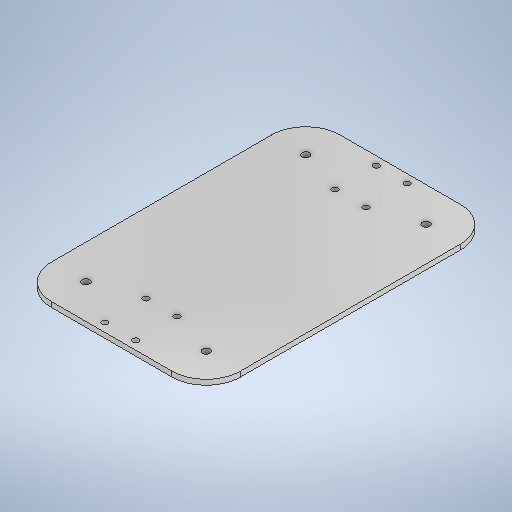
# Autodesk Inventor part: BedHousingFrame
Saved by Autodesk Inventor 2025.2 (Build 292293000, 293)
## iProperties
Created: 2025-05-31
Part Number: BedHousingFrame
Material: Generic
Document SubType Name: Modeling
Designer: Simon
Density: 1 g/cm^3
Appearance: Aluminum - Polished
Author: Simon
Autodesk Inventor part; units mm, degrees
ref_plane "YZ Plane" through (0, 0, 0) normal (1, 0, 0) x (0, 1, 0)
ref_plane "XZ Plane" through (0, 0, 0) normal (0, 1, 0) x (-1, 0, 0)
ref_plane "XY Plane" through (0, 0, 0) normal (0, 0, 1) x (1, 0, 0)
sketch "Sketch1" plane through (0, 0, 0) normal (0, 1, 0) x (-1, 0, 0)
  line L0 (-15, 33) -> (95, 33)
  line L1 (95, 33) -> (95, -135)
  line L2 (95, -135) -> (-15, -135)
  line L3 (-15, -135) -> (-15, 33)
  line L4 (95, 33) -> (95, 15)
  line L5 (-15, 33) -> (-15, 13)
  line L6 (95, -135) -> (95, -115)
  line L7 (-15, -135) -> (-15, -115)
  line L8 (40, -135) -> (40, -130)
  line L9 (31, -130) -> (49, -130)
  line L10 (49, -130) -> (49, -106)
  line L11 (49, -106) -> (31, -106)
  line L12 (31, -106) -> (31, -130)
  line L13 (40, 33) -> (40, 28)
  line L14 (31, 28) -> (49, 28)
  line L15 (49, 28) -> (49, 4)
  line L16 (49, 4) -> (31, 4)
  line L17 (31, 4) -> (31, 28)
  point P0 (0, 0)
  point P1 (47.5, 33)
  point P2 (12.5, 33)
  point P3 (67.5, -135)
  point P4 (32.5, -135)
  dimension "d4" = 110
  dimension "d5" = 168
  dimension "d22" = 5
  dimension "d23" = 18
  dimension "d24" = 24
  dimension "d25" = 5
  dimension "d26" = 18
  dimension "d27" = 24
  constraints: 36 end point, 7 perpendicular, 7 point on line, 4 midpoint, 2 horizontal, 2 parallel, 2 vertical
  measures "d4" distance of L1.end L2.end
  measures "d5" distance of L0.end L1.end
  measures "d22" distance of L8.start L8.end
  measures "d23" distance of L9.start L9.end
  measures "d24" distance of L9.end L10.end
  measures "d25" distance of L13.start L13.end
  measures "d26" distance of L14.start L14.end
  measures "d27" distance of L14.end L15.end
extrude "Extrusion2" add sketch "Sketch1" along normal blind 3 contours L0 L1 L2 L3 | L12 L11 L10 L9 | L14 L15 L16 L17
hole "Hole1" at (-49, 0, 28) at (-49, 0, 4) at (-31, 0, 28) at (-31, 0, 4) at (-49, 0, -130) at (-31, 0, -130) at (-31, 0, -106) at (-49, 0, -106) direction (0, -1, 0) diameter 3.4 end through all both
fillet "Fillet1" radius 20 4 edges at (15, 1.5, 33) (-95, 1.5, 33) (15, 1.5, -135) (-95, 1.5, -135)
ref_plane "Work Plane1" through (-75, 0, -51) normal (0, 0, 1) x (1, 0, 0)
ref_plane "Work Plane2" through (-40, 0, 13) normal (1, 0, 0) x (0, 0, -1)
sketch "Sketch2" plane through (0, 3, 0) normal (0, 1, 0) x (1, 0, 0)
  arc A0 (-95, -13) -> (-75, -33) centre (-75, -13) ccw projected
  line L0 (-95, -33) -> (-95, -13)
  line L1 (-75, -33) -> (-5, -33) projected
  line L2 (-95, -33) -> (-75, -33)
  line L3 (-75, -33) -> (-75, -13)
  line L4 (-75, -13) -> (-95, -13)
  arc A1 (-5, -33) -> (15, -13) centre (-5, -13) ccw projected
  line L5 (15, -33) -> (-5, -33)
  line L6 (15, -33) -> (15, -13)
  line L7 (-5, -33) -> (-5, -13)
  line L8 (-5, -13) -> (15, -13)
  arc A2 (15, 115) -> (-5, 135) centre (-5, 115) ccw projected
  line L9 (15, 135) -> (15, 115)
  line L10 (15, 135) -> (-5, 135)
  line L11 (-5, 135) -> (-5, 115)
  line L12 (-5, 115) -> (15, 115)
  arc A3 (-75, 135) -> (-95, 115) centre (-75, 115) ccw projected
  line L13 (-95, 135) -> (-95, 115)
  line L14 (-95, 135) -> (-75, 135)
  line L15 (-95, 115) -> (-95, -13) projected
  line L16 (-95, 115) -> (-75, 115)
  line L17 (-75, 115) -> (-75, 135)
  point P0 (0, 0)
  constraints: 32 end point, 7 tangent, 6 vertical, 5 perpendicular, 4 horizontal, 1 collinear, 1 point on line
hole "Hole2" at (-75, 3, 13) at (-75, 3, -115) at (-5, 3, -115) at (-5, 3, 13) direction (0, -1, 0) diameter 4.3 end through all
body "Solid1"
